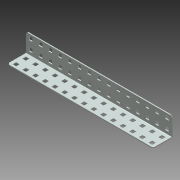
# Autodesk Inventor part: 276-2161
Saved by Autodesk Inventor 2013 (Build 170138000, 138)
## iProperties
Company: Autodesk Inc.
Category: Structure
Part Number: 276-2161
Document SubType Name: Sheet Metal
Designer: Autodesk Inc.
Density: 7.85 g/cm^3
Sheet Metal Rule: Default
Material: Steel
Mass: 80.2693 g
Surface Area: 180.989 cm^2
Volume: 10.2254 cm^3
Created: 2012-04-11
Catalog Web Link: http://www.vexrobotics.com/276-2161.html
Vendor: VEX
Author: Autodesk Inc.
Autodesk Inventor part; units mm, degrees
ref_plane "YZ Plane" through (0, 0, 0) normal (1, 0, 0) x (0, 1, 0)
ref_plane "XZ Plane" through (0, 0, 0) normal (0, 1, 0) x (-1, 0, 0)
ref_plane "XY Plane" through (0, 0, 0) normal (0, 0, 1) x (1, 0, 0)
sketch "Sketch1" plane through (0, 0, 0) normal (0, 0, 1) x (1, 0, 0)
  line L0 (-40.3471, 14.7344) -> (150.1529, 14.7344)
  line L1 (150.1529, 14.7344) -> (150.1529, -9.3956)
  line L2 (150.1529, -9.3956) -> (-40.3471, -9.3956)
  line L3 (-40.3471, -9.3956) -> (-40.3471, 14.7344)
  line L4 (-36.2831, 11.9404) -> (-31.7111, 11.9404)
  line L5 (-31.7111, 11.9404) -> (-31.7111, 7.3684)
  line L6 (-31.7111, 7.3684) -> (-36.2831, 7.3684)
  line L7 (-36.2831, 7.3684) -> (-36.2831, 11.9404)
  line L8 (-36.2831, -0.7596) -> (-31.7111, -0.7596)
  line L9 (-31.7111, -0.7596) -> (-31.7111, -5.3316)
  line L10 (-31.7111, -5.3316) -> (-36.2831, -5.3316)
  line L11 (-36.2831, -5.3316) -> (-36.2831, -0.7596)
  line L12 (-23.5831, 11.9404) -> (-19.0111, 11.9404)
  line L13 (-19.0111, 11.9404) -> (-19.0111, 7.3684)
  line L14 (-19.0111, 7.3684) -> (-23.5831, 7.3684)
  line L15 (-23.5831, 7.3684) -> (-23.5831, 11.9404)
  line L16 (-23.5831, -0.7596) -> (-19.0111, -0.7596)
  line L17 (-19.0111, -0.7596) -> (-19.0111, -5.3316)
  line L18 (-19.0111, -5.3316) -> (-23.5831, -5.3316)
  line L19 (-23.5831, -5.3316) -> (-23.5831, -0.7596)
  line L20 (-10.8831, 11.9404) -> (-6.3111, 11.9404)
  line L21 (-6.3111, 11.9404) -> (-6.3111, 7.3684)
  line L22 (-6.3111, 7.3684) -> (-10.8831, 7.3684)
  line L23 (-10.8831, 7.3684) -> (-10.8831, 11.9404)
  line L24 (-10.8831, -0.7596) -> (-6.3111, -0.7596)
  line L25 (-6.3111, -0.7596) -> (-6.3111, -5.3316)
  line L26 (-6.3111, -5.3316) -> (-10.8831, -5.3316)
  line L27 (-10.8831, -5.3316) -> (-10.8831, -0.7596)
  line L28 (1.8169, 11.9404) -> (6.3889, 11.9404)
  line L29 (6.3889, 11.9404) -> (6.3889, 7.3684)
  line L30 (6.3889, 7.3684) -> (1.8169, 7.3684)
  line L31 (1.8169, 7.3684) -> (1.8169, 11.9404)
  line L32 (1.8169, -0.7596) -> (6.3889, -0.7596)
  line L33 (6.3889, -0.7596) -> (6.3889, -5.3316)
  line L34 (6.3889, -5.3316) -> (1.8169, -5.3316)
  line L35 (1.8169, -5.3316) -> (1.8169, -0.7596)
  line L36 (14.5169, 11.9404) -> (19.0889, 11.9404)
  line L37 (19.0889, 11.9404) -> (19.0889, 7.3684)
  line L38 (19.0889, 7.3684) -> (14.5169, 7.3684)
  line L39 (14.5169, 7.3684) -> (14.5169, 11.9404)
  line L40 (14.5169, -0.7596) -> (19.0889, -0.7596)
  line L41 (19.0889, -0.7596) -> (19.0889, -5.3316)
  line L42 (19.0889, -5.3316) -> (14.5169, -5.3316)
  line L43 (14.5169, -5.3316) -> (14.5169, -0.7596)
  line L44 (27.2169, 11.9404) -> (31.7889, 11.9404)
  line L45 (31.7889, 11.9404) -> (31.7889, 7.3684)
  line L46 (31.7889, 7.3684) -> (27.2169, 7.3684)
  line L47 (27.2169, 7.3684) -> (27.2169, 11.9404)
  line L48 (27.2169, -0.7596) -> (31.7889, -0.7596)
  line L49 (31.7889, -0.7596) -> (31.7889, -5.3316)
  line L50 (31.7889, -5.3316) -> (27.2169, -5.3316)
  line L51 (27.2169, -5.3316) -> (27.2169, -0.7596)
  line L52 (39.9169, 11.9404) -> (44.4889, 11.9404)
  line L53 (44.4889, 11.9404) -> (44.4889, 7.3684)
  line L54 (44.4889, 7.3684) -> (39.9169, 7.3684)
  line L55 (39.9169, 7.3684) -> (39.9169, 11.9404)
  line L56 (39.9169, -0.7596) -> (44.4889, -0.7596)
  line L57 (44.4889, -0.7596) -> (44.4889, -5.3316)
  line L58 (44.4889, -5.3316) -> (39.9169, -5.3316)
  line L59 (39.9169, -5.3316) -> (39.9169, -0.7596)
  line L60 (52.6169, 11.9404) -> (57.1889, 11.9404)
  line L61 (57.1889, 11.9404) -> (57.1889, 7.3684)
  line L62 (57.1889, 7.3684) -> (52.6169, 7.3684)
  line L63 (52.6169, 7.3684) -> (52.6169, 11.9404)
  line L64 (52.6169, -0.7596) -> (57.1889, -0.7596)
  line L65 (57.1889, -0.7596) -> (57.1889, -5.3316)
  line L66 (57.1889, -5.3316) -> (52.6169, -5.3316)
  line L67 (52.6169, -5.3316) -> (52.6169, -0.7596)
  line L68 (65.3169, 11.9404) -> (69.8889, 11.9404)
  line L69 (69.8889, 11.9404) -> (69.8889, 7.3684)
  line L70 (69.8889, 7.3684) -> (65.3169, 7.3684)
  line L71 (65.3169, 7.3684) -> (65.3169, 11.9404)
  line L72 (65.3169, -0.7596) -> (69.8889, -0.7596)
  line L73 (69.8889, -0.7596) -> (69.8889, -5.3316)
  line L74 (69.8889, -5.3316) -> (65.3169, -5.3316)
  line L75 (65.3169, -5.3316) -> (65.3169, -0.7596)
  line L76 (78.0169, 11.9404) -> (82.5889, 11.9404)
  line L77 (82.5889, 11.9404) -> (82.5889, 7.3684)
  line L78 (82.5889, 7.3684) -> (78.0169, 7.3684)
  line L79 (78.0169, 7.3684) -> (78.0169, 11.9404)
  line L80 (78.0169, -0.7596) -> (82.5889, -0.7596)
  line L81 (82.5889, -0.7596) -> (82.5889, -5.3316)
  line L82 (82.5889, -5.3316) -> (78.0169, -5.3316)
  line L83 (78.0169, -5.3316) -> (78.0169, -0.7596)
  line L84 (90.7169, 11.9404) -> (95.2889, 11.9404)
  line L85 (95.2889, 11.9404) -> (95.2889, 7.3684)
  line L86 (95.2889, 7.3684) -> (90.7169, 7.3684)
  line L87 (90.7169, 7.3684) -> (90.7169, 11.9404)
  line L88 (90.7169, -0.7596) -> (95.2889, -0.7596)
  line L89 (95.2889, -0.7596) -> (95.2889, -5.3316)
  line L90 (95.2889, -5.3316) -> (90.7169, -5.3316)
  line L91 (90.7169, -5.3316) -> (90.7169, -0.7596)
  line L92 (103.4169, 11.9404) -> (107.9889, 11.9404)
  line L93 (107.9889, 11.9404) -> (107.9889, 7.3684)
  line L94 (107.9889, 7.3684) -> (103.4169, 7.3684)
  line L95 (103.4169, 7.3684) -> (103.4169, 11.9404)
  line L96 (103.4169, -0.7596) -> (107.9889, -0.7596)
  line L97 (107.9889, -0.7596) -> (107.9889, -5.3316)
  line L98 (107.9889, -5.3316) -> (103.4169, -5.3316)
  line L99 (103.4169, -5.3316) -> (103.4169, -0.7596)
  line L100 (116.1169, 11.9404) -> (120.6889, 11.9404)
  line L101 (120.6889, 11.9404) -> (120.6889, 7.3684)
  line L102 (120.6889, 7.3684) -> (116.1169, 7.3684)
  line L103 (116.1169, 7.3684) -> (116.1169, 11.9404)
  line L104 (116.1169, -0.7596) -> (120.6889, -0.7596)
  line L105 (120.6889, -0.7596) -> (120.6889, -5.3316)
  line L106 (120.6889, -5.3316) -> (116.1169, -5.3316)
  line L107 (116.1169, -5.3316) -> (116.1169, -0.7596)
  line L108 (128.8169, 11.9404) -> (133.3889, 11.9404)
  line L109 (133.3889, 11.9404) -> (133.3889, 7.3684)
  line L110 (133.3889, 7.3684) -> (128.8169, 7.3684)
  line L111 (128.8169, 7.3684) -> (128.8169, 11.9404)
  line L112 (128.8169, -0.7596) -> (133.3889, -0.7596)
  line L113 (133.3889, -0.7596) -> (133.3889, -5.3316)
  line L114 (133.3889, -5.3316) -> (128.8169, -5.3316)
  line L115 (128.8169, -5.3316) -> (128.8169, -0.7596)
  line L116 (141.5169, 11.9404) -> (146.0889, 11.9404)
  line L117 (146.0889, 11.9404) -> (146.0889, 7.3684)
  line L118 (146.0889, 7.3684) -> (141.5169, 7.3684)
  line L119 (141.5169, 7.3684) -> (141.5169, 11.9404)
  line L120 (141.5169, -0.7596) -> (146.0889, -0.7596)
  line L121 (146.0889, -0.7596) -> (146.0889, -5.3316)
  line L122 (146.0889, -5.3316) -> (141.5169, -5.3316)
  line L123 (141.5169, -5.3316) -> (141.5169, -0.7596)
  dimension "d0" = 2.794
  dimension "d1" = 8.128
  dimension "d2" = 4.572
  dimension "d3" = 4.572
  dimension "d4" = 4.572
  dimension "d5" = 24.13
  dimension "d8" = 12.7
  dimension "d13" = 4.064
  dimension "d31" = 4.064
  measures "d0" distance between parallel lines of L0 L4
  measures "d1" distance between parallel lines of L6 L8
  measures "d2" distance of L6.end L4.start
  measures "d3" distance of L10.end L8.start
  measures "d4" distance of L4.start L4.end
  measures "d5" distance of L2.end L0.start
  measures "d8" distance of L4.end L13.start
  measures "d13" distance between parallel lines of L1 L117
  measures "d31" distance between parallel lines of L7 L3
extrude "Plate1" add sketch "Sketch1" along normal blind 1.27
sketch "Sketch2" plane through (150.1529, -9.3956, 1.27) normal (0, 1, 0) x (-1, 0, 0)
  line L0 (0, 0) -> (190.5, 0)
  line L1 (190.5, 0) -> (190.5, 24.13)
  line L2 (190.5, 24.13) -> (0, 24.13)
  line L3 (0, 24.13) -> (0, 0)
  constraints: 6 end point, 1 horizontal, 1 perpendicular, 1 vertical
sheet face with bend "Flange1" sketch "Sketch2" thickness 1.27 toward (0, -1, 0) bend radius 0.8636 relief straight relief width 1.27 relief depth 0.635
bend "Bend1"
chamfer "Corner Chamfer1" distance 1.905 angle 45 4 edges at (-40.3471, 14.7344, 0.635) (-40.3471, -10.0306, 25.4) (150.1529, -10.0306, 25.4) (150.1529, 14.7344, 0.635)
sketch "Sketch3" plane through (-40.3471, -9.3956, 2.1336) normal (0, 1, 0) x (1, 0, 0)
  line L0 (0, 0) -> (0, -21.3614) projected
  line L1 (1.905, -23.2664) -> (188.595, -23.2664) projected
  line L2 (4.064, -15.9004) -> (8.636, -15.9004)
  line L3 (8.636, -15.9004) -> (8.636, -20.4724)
  line L4 (8.636, -20.4724) -> (4.064, -20.4724)
  line L5 (4.064, -20.4724) -> (4.064, -15.9004)
  line L6 (4.064, -3.2004) -> (8.636, -3.2004)
  line L7 (8.636, -3.2004) -> (8.636, -7.7724)
  line L8 (8.636, -7.7724) -> (4.064, -7.7724)
  line L9 (4.064, -7.7724) -> (4.064, -3.2004)
  line L10 (16.764, -15.9004) -> (21.336, -15.9004)
  line L11 (21.336, -15.9004) -> (21.336, -20.4724)
  line L12 (21.336, -20.4724) -> (16.764, -20.4724)
  line L13 (16.764, -20.4724) -> (16.764, -15.9004)
  line L14 (16.764, -3.2004) -> (21.336, -3.2004)
  line L15 (21.336, -3.2004) -> (21.336, -7.7724)
  line L16 (21.336, -7.7724) -> (16.764, -7.7724)
  line L17 (16.764, -7.7724) -> (16.764, -3.2004)
  line L18 (29.464, -15.9004) -> (34.036, -15.9004)
  line L19 (34.036, -15.9004) -> (34.036, -20.4724)
  line L20 (34.036, -20.4724) -> (29.464, -20.4724)
  line L21 (29.464, -20.4724) -> (29.464, -15.9004)
  line L22 (29.464, -3.2004) -> (34.036, -3.2004)
  line L23 (34.036, -3.2004) -> (34.036, -7.7724)
  line L24 (34.036, -7.7724) -> (29.464, -7.7724)
  line L25 (29.464, -7.7724) -> (29.464, -3.2004)
  line L26 (42.164, -15.9004) -> (46.736, -15.9004)
  line L27 (46.736, -15.9004) -> (46.736, -20.4724)
  line L28 (46.736, -20.4724) -> (42.164, -20.4724)
  line L29 (42.164, -20.4724) -> (42.164, -15.9004)
  line L30 (42.164, -3.2004) -> (46.736, -3.2004)
  line L31 (46.736, -3.2004) -> (46.736, -7.7724)
  line L32 (46.736, -7.7724) -> (42.164, -7.7724)
  line L33 (42.164, -7.7724) -> (42.164, -3.2004)
  line L34 (54.864, -15.9004) -> (59.436, -15.9004)
  line L35 (59.436, -15.9004) -> (59.436, -20.4724)
  line L36 (59.436, -20.4724) -> (54.864, -20.4724)
  line L37 (54.864, -20.4724) -> (54.864, -15.9004)
  line L38 (54.864, -3.2004) -> (59.436, -3.2004)
  line L39 (59.436, -3.2004) -> (59.436, -7.7724)
  line L40 (59.436, -7.7724) -> (54.864, -7.7724)
  line L41 (54.864, -7.7724) -> (54.864, -3.2004)
  line L42 (67.564, -15.9004) -> (72.136, -15.9004)
  line L43 (72.136, -15.9004) -> (72.136, -20.4724)
  line L44 (72.136, -20.4724) -> (67.564, -20.4724)
  line L45 (67.564, -20.4724) -> (67.564, -15.9004)
  line L46 (67.564, -3.2004) -> (72.136, -3.2004)
  line L47 (72.136, -3.2004) -> (72.136, -7.7724)
  line L48 (72.136, -7.7724) -> (67.564, -7.7724)
  line L49 (67.564, -7.7724) -> (67.564, -3.2004)
  line L50 (80.264, -15.9004) -> (84.836, -15.9004)
  line L51 (84.836, -15.9004) -> (84.836, -20.4724)
  line L52 (84.836, -20.4724) -> (80.264, -20.4724)
  line L53 (80.264, -20.4724) -> (80.264, -15.9004)
  line L54 (80.264, -3.2004) -> (84.836, -3.2004)
  line L55 (84.836, -3.2004) -> (84.836, -7.7724)
  line L56 (84.836, -7.7724) -> (80.264, -7.7724)
  line L57 (80.264, -7.7724) -> (80.264, -3.2004)
  line L58 (92.964, -15.9004) -> (97.536, -15.9004)
  line L59 (97.536, -15.9004) -> (97.536, -20.4724)
  line L60 (97.536, -20.4724) -> (92.964, -20.4724)
  line L61 (92.964, -20.4724) -> (92.964, -15.9004)
  line L62 (92.964, -3.2004) -> (97.536, -3.2004)
  line L63 (97.536, -3.2004) -> (97.536, -7.7724)
  line L64 (97.536, -7.7724) -> (92.964, -7.7724)
  line L65 (92.964, -7.7724) -> (92.964, -3.2004)
  line L66 (105.664, -15.9004) -> (110.236, -15.9004)
  line L67 (110.236, -15.9004) -> (110.236, -20.4724)
  line L68 (110.236, -20.4724) -> (105.664, -20.4724)
  line L69 (105.664, -20.4724) -> (105.664, -15.9004)
  line L70 (105.664, -3.2004) -> (110.236, -3.2004)
  line L71 (110.236, -3.2004) -> (110.236, -7.7724)
  line L72 (110.236, -7.7724) -> (105.664, -7.7724)
  line L73 (105.664, -7.7724) -> (105.664, -3.2004)
  line L74 (118.364, -15.9004) -> (122.936, -15.9004)
  line L75 (122.936, -15.9004) -> (122.936, -20.4724)
  line L76 (122.936, -20.4724) -> (118.364, -20.4724)
  line L77 (118.364, -20.4724) -> (118.364, -15.9004)
  line L78 (118.364, -3.2004) -> (122.936, -3.2004)
  line L79 (122.936, -3.2004) -> (122.936, -7.7724)
  line L80 (122.936, -7.7724) -> (118.364, -7.7724)
  line L81 (118.364, -7.7724) -> (118.364, -3.2004)
  line L82 (131.064, -15.9004) -> (135.636, -15.9004)
  line L83 (135.636, -15.9004) -> (135.636, -20.4724)
  line L84 (135.636, -20.4724) -> (131.064, -20.4724)
  line L85 (131.064, -20.4724) -> (131.064, -15.9004)
  line L86 (131.064, -3.2004) -> (135.636, -3.2004)
  line L87 (135.636, -3.2004) -> (135.636, -7.7724)
  line L88 (135.636, -7.7724) -> (131.064, -7.7724)
  line L89 (131.064, -7.7724) -> (131.064, -3.2004)
  line L90 (143.764, -15.9004) -> (148.336, -15.9004)
  line L91 (148.336, -15.9004) -> (148.336, -20.4724)
  line L92 (148.336, -20.4724) -> (143.764, -20.4724)
  line L93 (143.764, -20.4724) -> (143.764, -15.9004)
  line L94 (143.764, -3.2004) -> (148.336, -3.2004)
  line L95 (148.336, -3.2004) -> (148.336, -7.7724)
  line L96 (148.336, -7.7724) -> (143.764, -7.7724)
  line L97 (143.764, -7.7724) -> (143.764, -3.2004)
  line L98 (156.464, -15.9004) -> (161.036, -15.9004)
  line L99 (161.036, -15.9004) -> (161.036, -20.4724)
  line L100 (161.036, -20.4724) -> (156.464, -20.4724)
  line L101 (156.464, -20.4724) -> (156.464, -15.9004)
  line L102 (156.464, -3.2004) -> (161.036, -3.2004)
  line L103 (161.036, -3.2004) -> (161.036, -7.7724)
  line L104 (161.036, -7.7724) -> (156.464, -7.7724)
  line L105 (156.464, -7.7724) -> (156.464, -3.2004)
  line L106 (169.164, -15.9004) -> (173.736, -15.9004)
  line L107 (173.736, -15.9004) -> (173.736, -20.4724)
  line L108 (173.736, -20.4724) -> (169.164, -20.4724)
  line L109 (169.164, -20.4724) -> (169.164, -15.9004)
  line L110 (169.164, -3.2004) -> (173.736, -3.2004)
  line L111 (173.736, -3.2004) -> (173.736, -7.7724)
  line L112 (173.736, -7.7724) -> (169.164, -7.7724)
  line L113 (169.164, -7.7724) -> (169.164, -3.2004)
  line L114 (181.864, -15.9004) -> (186.436, -15.9004)
  line L115 (186.436, -15.9004) -> (186.436, -20.4724)
  line L116 (186.436, -20.4724) -> (181.864, -20.4724)
  line L117 (181.864, -20.4724) -> (181.864, -15.9004)
  line L118 (181.864, -3.2004) -> (186.436, -3.2004)
  line L119 (186.436, -3.2004) -> (186.436, -7.7724)
  line L120 (186.436, -7.7724) -> (181.864, -7.7724)
  line L121 (181.864, -7.7724) -> (181.864, -3.2004)
  dimension "d25" = 4.572
  dimension "d26" = 4.572
  dimension "d27" = 8.128
  dimension "d28" = 4.064
  dimension "d29" = 2.794
  dimension "d30" = 4.572
  dimension "d34" = 12.7
  constraints: 240 end point, 4 parallel, 3 horizontal, 2 perpendicular, 1 collinear, 224 other
  measures "d25" distance of L8.end L6.start
  measures "d26" distance of L4.end L2.start
  measures "d27" distance between parallel lines of L8 L2
  measures "d28" distance between parallel lines of L0 L9
  measures "d29" distance between parallel lines of L1 L4
  measures "d30" distance of L3.end L4.end
  measures "d34" distance of L8.end L17.start
extrude "Cut1" cut sketch "Sketch3" against normal blind 1.27
sketch "Sketch4" plane through (-40.3471, -8.532, 1.27) normal (0, 0, 1) x (1, 0, 0)
  line L0 (8.636, 20.4724) -> (8.636, 15.9004) projected
  line L1 (8.636, 15.9004) -> (4.064, 15.9004) projected
  line L2 (4.064, 15.9004) -> (4.064, 20.4724) projected
  line L3 (4.064, 20.4724) -> (8.636, 20.4724) projected
  circle A0 centre (6.35, 18.1864) radius 2.286
  point P0 (40.3471, 8.532)
  constraints: 4 tangent, 1 centre point
surface extrude "ExtrusionSrf1" sketch "Sketch4" against normal up to surface (1.27 mm away) shown no curves A0
pattern_linear "Rectangular Pattern1" count 15 spacing 12.7 along (1, 0, 0) count 2 spacing 12.7 along (0, -1, 0) of "ExtrusionSrf1"
sketch "Sketch5" plane through (-40.3471, -9.3956, 2.1336) normal (0, 1, 0) x (1, 0, 0)
  line L0 (4.064, -20.4724) -> (4.064, -15.9004) projected
  line L1 (4.064, -15.9004) -> (8.636, -15.9004) projected
  line L2 (8.636, -15.9004) -> (8.636, -20.4724) projected
  line L3 (8.636, -20.4724) -> (4.064, -20.4724) projected
  circle A0 centre (6.35, -18.1864) radius 2.286
  point P0 (40.3471, 2.1336)
  constraints: 4 tangent, 1 centre point
surface extrude "ExtrusionSrf31" sketch "Sketch5" against normal up to surface (1.27 mm away) shown no curves A0
pattern_linear "Rectangular Pattern2" count 15 spacing 12.7 along (1, 0, 0) count 2 spacing 12.7 along (0, 0, -1) of "ExtrusionSrf31"
equation "\"d39\" = Thickness"
equation "\"d15\" = BendReliefWidth"
equation "\"d17\" = MinimumRemnant"
equation "\"d21\" = BendRadius"
equation "\"d16\" = BendReliefDepth"
equation "\"d18\" = BendRadius"
equation "\"BendReliefWidth\" = Thickness"
equation "\"BendReliefDepth\" = 0.5 * Thickness"
equation "\"CornerReliefSize\" = 4 * Thickness"
equation "\"MinimumRemnant\" = 2 * Thickness"
equation "\"TransitionRadius\" = BendRadius"
equation "\"d14\" = BendRadius"
equation "\"JacobiRadiusSize\" = Thickness"
equation "\"GapSize\" = Thickness"
equation "\"Thickness\" = 1.27"
equation "\"BendRadius\" = 0.8636"
body "Solid1"
body "Srf1"
body "Srf2"
body "Srf3"
body "Srf4"
body "Srf5"
body "Srf6"
body "Srf7"
body "Srf8"
body "Srf9"
body "Srf10"
body "Srf11"
body "Srf12"
body "Srf13"
body "Srf14"
body "Srf15"
body "Srf16"
body "Srf17"
body "Srf18"
body "Srf19"
body "Srf20"
body "Srf21"
body "Srf22"
body "Srf23"
body "Srf24"
body "Srf25"
body "Srf26"
body "Srf27"
body "Srf28"
body "Srf29"
body "Srf30"
body "Srf31"
body "Srf32"
body "Srf33"
body "Srf34"
body "Srf35"
body "Srf36"
body "Srf37"
body "Srf38"
body "Srf39"
body "Srf40"
body "Srf41"
body "Srf42"
body "Srf43"
body "Srf44"
body "Srf45"
body "Srf46"
body "Srf47"
body "Srf48"
body "Srf49"
body "Srf50"
body "Srf51"
body "Srf52"
body "Srf53"
body "Srf54"
body "Srf55"
body "Srf56"
body "Srf57"
body "Srf58"
body "Srf59"
body "Srf60"
